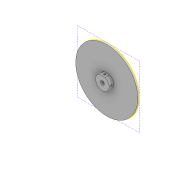
# Autodesk Inventor part: wheel
Saved by Autodesk Inventor 2020 (Build 240168000, 168)
## iProperties
Created: 2021-06-14
Part Number: wheel
Material: Generic
Document SubType Name: Modeling
Designer: Aidan Lee
Density: 1 g/cm^3
Appearance: Default
Author: Aidan Lee
Autodesk Inventor part; units mm, degrees
ref_plane "YZ Plane" through (0, 0, 0) normal (1, 0, 0) x (0, 1, 0)
ref_plane "XZ Plane" through (0, 0, 0) normal (0, 1, 0) x (-1, 0, 0)
ref_plane "XY Plane" through (0, 0, 0) normal (0, 0, 1) x (1, 0, 0)
sketch "Sketch1" plane through (0, 0, 0) normal (0, 0, 1) x (1, 0, 0)
  spline S0 degree 3 poles (-8.9262, 55.5372) (-8.7839, 55.3802) (-8.4991, 55.0662) (-8.0852, 54.5835) (-7.6813, 54.0924) (-7.2889, 53.592) (-6.9084, 53.0826) (-6.5406, 52.5638) (-6.1865, 52.0357) (-5.8469, 51.4981) (-5.5231, 50.9508) (-5.2164, 50.3937) (-4.9286, 49.8267) (-4.6617, 49.2495) (-4.4187, 48.6617) (-4.2033, 48.0633) (-4.0539, 47.5547) (-3.9553, 47.1422) (-3.9241, 46.9325) (-3.9085, 46.8277) knots 0 0 0 0 0.063581 0.127162 0.190743 0.254324 0.317905 0.381486 0.445066 0.508647 0.572227 0.635807 0.699386 0.762964 0.826542 0.890117 0.953687 0.985476 1.017256 1.017256 1.017256 1.017256
  spline S1 degree 3 poles (-3.9085, 46.8277) (-3.8988, 46.6849) (-3.8795, 46.3993) (-3.8286, 45.9728) (-3.7545, 45.5498) (-3.6583, 45.1311) (-3.5319, 44.7205) (-3.3763, 44.3201) (-3.189, 43.9333) (-2.9645, 43.5666) (-2.7433, 43.2845) (-2.5493, 43.0739) (-2.3922, 42.9274) (-2.2262, 42.7911) (-2.0526, 42.6646) (-1.8686, 42.5537) (-1.678, 42.4548) (-1.4812, 42.3683) (-1.2769, 42.302) (-1.0697, 42.2449) (-0.8577, 42.21) (-0.6441, 42.187) (-0.3577, 42.1846) (0, 42.1894) (0.3577, 42.1846) (0.6441, 42.187) (0.8577, 42.21) (1.0697, 42.2449) (1.2769, 42.302) (1.4812, 42.3683) (1.678, 42.4548) (1.8686, 42.5537) (2.0526, 42.6646) (2.2262, 42.7911) (2.3922, 42.9274) (2.5493, 43.0739) (2.7433, 43.2845) (2.9645, 43.5666) (3.189, 43.9333) (3.3763, 44.3201) (3.5319, 44.7205) (3.6583, 45.1311) (3.7545, 45.5498) (3.8286, 45.9728) (3.8795, 46.3993) (3.8988, 46.6849) (3.9085, 46.8277) knots 0 0 0 0 0.04293 0.085861 0.12879 0.17172 0.214646 0.257562 0.300476 0.343394 0.386302 0.407769 0.429238 0.450698 0.472163 0.49363 0.515088 0.536554 0.558017 0.579478 0.600945 0.622403 0.64387 0.686802 0.729734 0.751201 0.772659 0.794126 0.815587 0.83705 0.858516 0.879974 0.901441 0.922906 0.944366 0.965835 0.987302 1.03021 1.073128 1.116042 1.158958 1.201884 1.244814 1.287743 1.330674 1.373604 1.373604 1.373604 1.373604
  spline S2 degree 3 poles (3.9085, 46.8277) (3.9241, 46.9325) (3.9553, 47.1422) (4.0539, 47.5547) (4.2033, 48.0633) (4.4187, 48.6617) (4.6617, 49.2495) (4.9286, 49.8267) (5.2164, 50.3937) (5.5231, 50.9508) (5.8469, 51.4981) (6.1865, 52.0357) (6.5406, 52.5638) (6.9084, 53.0826) (7.2889, 53.592) (7.6813, 54.0924) (8.0852, 54.5835) (8.4991, 55.0662) (8.7839, 55.3802) (8.9262, 55.5372) knots 0 0 0 0 0.03178 0.063568 0.127139 0.190714 0.254291 0.31787 0.381449 0.445029 0.508609 0.572189 0.63577 0.699351 0.762932 0.826513 0.890094 0.953675 1.017256 1.017256 1.017256 1.017256
  circle A0 centre (0, 0) radius 42.1875 construction
  circle A1 centre (0, 0) radius 46.9846 construction
  circle A2 centre (0, 0) radius 50 construction
  circle A3 centre (0, 0) radius 56.25
  point P0 (-8.5013, 55.0643)
  point P1 (-8.0869, 54.5821)
  point P2 (-7.6832, 54.0908)
  point P3 (-7.2909, 53.5905)
  point P4 (-6.9105, 53.081)
  point P5 (-6.5429, 52.5623)
  point P6 (-6.1889, 52.0341)
  point P7 (-5.8496, 51.4965)
  point P8 (-5.526, 50.9492)
  point P9 (-5.2196, 50.3921)
  point P10 (-4.9321, 49.825)
  point P11 (-4.6657, 49.2477)
  point P12 (-4.4233, 48.6599)
  point P13 (-4.2093, 48.0613)
  point P14 (-4.031, 47.4511)
  point P15 (-3.9598, 47.1413)
  point P16 (-3.8758, 46.3996)
  point P17 (-3.8247, 45.9733)
  point P18 (-3.7508, 45.5505)
  point P19 (-3.6533, 45.1324)
  point P20 (-3.527, 44.7221)
  point P21 (-3.371, 44.3223)
  point P22 (-3.1828, 43.9367)
  point P23 (-2.9576, 43.5713)
  point P24 (-2.6935, 43.2332)
  point P25 (-2.5474, 43.0758)
  point P26 (-2.3907, 42.9291)
  point P27 (-2.225, 42.7928)
  point P28 (-2.0509, 42.6672)
  point P29 (-1.8675, 42.5557)
  point P30 (-1.677, 42.4569)
  point P31 (-1.48, 42.3717)
  point P32 (-1.2764, 42.3036)
  point P33 (-1.069, 42.2486)
  point P34 (-0.8574, 42.212)
  point P35 (-0.6439, 42.1905)
  point P36 (-0.4293, 42.1857)
  point P37 (0, 42.1875)
  point P38 (0.4293, 42.1857)
  point P39 (0.6439, 42.1905)
  point P40 (0.8574, 42.212)
  point P41 (1.069, 42.2486)
  point P42 (1.2764, 42.3036)
  point P43 (1.48, 42.3717)
  point P44 (1.677, 42.4569)
  point P45 (1.8675, 42.5557)
  point P46 (2.0509, 42.6672)
  point P47 (2.225, 42.7928)
  point P48 (2.3907, 42.9291)
  point P49 (2.5474, 43.0758)
  point P50 (2.6935, 43.2332)
  point P51 (2.9576, 43.5713)
  point P52 (3.1828, 43.9367)
  point P53 (3.371, 44.3223)
  point P54 (3.527, 44.7221)
  point P55 (3.6533, 45.1324)
  point P56 (3.7508, 45.5505)
  point P57 (3.8247, 45.9733)
  point P58 (3.8758, 46.3996)
  point P59 (3.9598, 47.1413)
  point P60 (4.031, 47.4511)
  point P61 (4.2093, 48.0613)
  point P62 (4.4233, 48.6599)
  point P63 (4.6657, 49.2477)
  point P64 (4.9321, 49.825)
  point P65 (5.2196, 50.3921)
  point P66 (5.526, 50.9492)
  point P67 (5.8496, 51.4965)
  point P68 (6.1889, 52.0341)
  point P69 (6.5429, 52.5623)
  point P70 (6.9105, 53.081)
  point P71 (7.2909, 53.5905)
  point P72 (7.6832, 54.0908)
  point P73 (8.0869, 54.5821)
  point P74 (8.5013, 55.0643)
  constraints: 4 centre point, 2 point on circle, 165 other
extrude "Extrusion1" add sketch "Sketch1" against normal blind 16
extrude "Extrusion2" cut sketch "Sketch1" against normal through all contours A3 S2 S1 S0 picked at (0.9155, 51.5438)
pattern_circular "Circular Pattern1" count 16 over 360 about axis through (0, 0, 0) along (0, 0, -1) of "Extrusion2"
sketch "Measuring" plane through (0, 0, -16) normal (0, 0, -1) x (-1, 0, 0)
  circle A0 centre (0, 0) radius 56.25 projected
  circle A1 centre (0, 0) radius 50
  circle A2 centre (73.063, 68.2774) radius 50 construction
  line L0 (27.9744, 52.4494) -> (54.2214, 24.3627) construction
  line L1 (41.0979, 38.406) -> (73.063, 68.2774) construction
  dimension "d37" = 100
  dimension "d45" = 6.25
  dimension "d46" = 100
  dimension "d47" = 43.75
  constraints: 4 end point, 2 centre point, 1 coincident, 1 equal radius, 1 midpoint, 1 perpendicular, 3 other
  measures "d37" diameter of A1
  measures "d46" diameter of A2
  measures "d47" distance from line of L1.end L0
sketch "Sketch11" plane through (0, 0, 0) normal (1, 0, 0) x (0, 1, 0)
  line L0 (13.8864, 0) -> (-13.8864, 0) construction
  line L1 (-13.8864, 0) -> (-13.8864, -7) construction
  line L2 (-13.8864, -7) -> (13.8864, -7) construction
  line L3 (13.8864, -7) -> (13.8864, 0) construction
  circle A0 centre (0, -3.5) radius 1.5 construction
  line L4 (-1.3941, -2) -> (1.3941, -2) construction
  line L5 (-3.9085, -16) -> (3.9085, -16) construction
  line L6 (-67.1444, 3.8787) -> (73.9482, 3.8787)
  line L7 (73.9482, 3.8787) -> (73.9482, -7)
  line L8 (73.9482, -7) -> (-67.1444, -7)
  line L9 (-67.1444, -7) -> (-67.1444, 3.8787)
  point P0 (0, 0)
  point P1 (0, 0)
  point P2 (-13.8864, -3.5)
  point P3 (0, -2)
  dimension "d48" = 3
  dimension "d49" = 2
  dimension "d50" = 9
  dimension "d58" = 7
  constraints: 18 end point, 4 parallel, 3 horizontal, 3 midpoint, 3 vertical alignment, 2 coincident, 2 perpendicular, 1 collinear, 1 horizontal alignment, 2 other
  measures "d49" distance between parallel lines of L0 L4
  measures "d50" distance between parallel lines of L5 L2
  measures "d58" distance of L2.end L0.start
extrude "Thinner" cut sketch "Sketch11" against normal through all both and the other way through all
sketch "Sketch12" plane through (-16.8651, 41.399, -7) normal (0, 0, 1) x (0.9476, 0.3195, 0)
  circle A0 centre (2.7546, -44.6175) radius 3
  dimension "d54" = 6
  constraints: 1 centre point, 1 coincident
  measures "d54" diameter of A0
extrude "Hole" cut sketch "Sketch12" against normal blind 20
sketch "Sketch13" plane through (-16.8651, 41.399, -7) normal (0, 0, 1) x (0.9476, 0.3195, 0)
  circle A0 centre (2.7546, -44.6175) radius 11
  circle A1 centre (2.7546, -44.6175) radius 3 projected
  dimension "d57" = 8
  constraints: 1 centre point, 1 coincident
  measures "d57" radial gap between concentric circles of A0 A1
extrude "Coupler" add sketch "Sketch13" along normal blind 7
sketch "Sketch14" plane through (-16.8651, 41.399, -7) normal (0, 0, 1) x (0.9476, 0.3195, 0)
  circle A0 centre (11.251, -19.4175) radius 9
  line L0 (16.2331, -4.641) -> (2.7546, -44.6175) construction
  circle A1 centre (2.7546, -44.6175) radius 11 construction
  circle A2 centre (2.7546, -44.6175) radius 11 construction
  line L1 (6.269, -34.194) -> (16.2331, -4.641) construction
  circle A3 centre (-14.821, -24.6594) radius 9
  circle A4 centre (-23.3174, -49.8593) radius 9
  circle A5 centre (-5.7418, -69.8174) radius 9
  circle A6 centre (20.3302, -64.5756) radius 9
  circle A7 centre (28.8266, -39.3756) radius 9
  dimension "d61" = 18
  dimension "d64" = 360
  constraints: 6 centre point, 4 end point, 2 point on line, 1 collinear, 1 midpoint, 15 other
  measures "d61" diameter of A0
extrude "Cutouts" cut sketch "Sketch14" against normal through all
sketch "Sketch15" plane through (0, 0, 0) normal (1, 0, 0) x (0, 1, 0)
  circle A0 centre (0, -3.5) radius 1.5
  line L0 (11, 0) -> (-11, 0) projected
  line L1 (0, 0) -> (0, -7) construction
  line L2 (0, -7) -> (0, 0) construction
  line L3 (-11, -7) -> (11, -7) construction
  point P0 (0, 0)
  point P1 (-10.9663, -7)
  dimension "d68" = 3
  constraints: 4 end point, 2 midpoint, 1 centre point, 1 coincident, 1 collinear, 1 horizontal alignment, 1 point on line, 1 vertical, 1 vertical alignment
  measures "d68" diameter of A0
extrude "SetScrewHole1" cut sketch "Sketch15" along normal through all
sketch "Sketch16" plane through (0, 0, 0) normal (0, 1, 0) x (-1, 0, 0)
  circle A0 centre (0, -3.5) radius 1.5
  line L0 (-11, -7) -> (11, -7) projected
  line L1 (0, 0) -> (0, -7) construction
  dimension "d71" = 3
  constraints: 2 end point, 2 midpoint, 1 centre point, 1 coincident, 1 vertical alignment
  measures "d71" diameter of A0
extrude "Extrusion14" cut sketch "Sketch16" along normal through all
thread "Thread3" size "M3x0.5" class "6H" standard "ANSI Metric M Profile" full length
thread "Thread4" size "M3x0.5" class "6H" standard "ANSI Metric M Profile" full length
sketch "Sketch17" plane through (-16.8651, 41.399, -7) normal (0, 0, 1) x (0.9476, 0.3195, 0)
  line L0 (-62.2572, 14.3784) -> (64.742, 14.3784)
  line L1 (64.742, 14.3784) -> (64.742, -104.7192)
  line L2 (64.742, -104.7192) -> (-62.2572, -104.7192)
  line L3 (-62.2572, -104.7192) -> (-62.2572, 14.3784)
  point P0 (2.7546, -44.6175)
  constraints: 8 end point, 2 parallel, 1 horizontal, 1 perpendicular
extrude "Extrusion15" cut sketch "Sketch17" against normal blind 10
sketch "Sketch18" plane through (0, 0, -7) normal (0, 0, -1) x (-1, 0, 0)
  circle A0 centre (0, 0) radius 50
  dimension "d80" = 100
  constraints: 1 centre point, 1 coincident
  measures "d80" diameter of A0
extrude "Extrusion16" add sketch "Sketch18" along normal blind 3
sketch "Sketch19" plane through (0, 0, -10) normal (0, 0, -1) x (-1, 0, 0)
  line L0 (-50, 50) -> (50, 50) construction
  line L1 (50, 50) -> (50, -50) construction
  line L2 (50, -50) -> (-50, -50) construction
  line L3 (-50, -50) -> (-50, 50) construction
  circle A0 centre (0, 0) radius 50 projected
  constraints: 2 tangent, 2 other
sketch "Sketch20" plane through (0, 0, 0) normal (1, 0, 0) x (0, 1, 0)
  line L0 (-50, -7) -> (50, -7) projected
  line L1 (18.4735, 2.9106) -> (10, 2.9106)
  line L2 (10, 2.9106) -> (10, -7)
  line L3 (10, -7) -> (18.4735, -7)
  line L4 (18.4735, -7) -> (18.4735, 2.9106)
  point P0 (0, 0)
  dimension "d124" = 10
  constraints: 8 end point, 2 parallel, 1 horizontal, 1 perpendicular, 1 point on line
  measures "d124" distance from line of point (0, 0) L2
extrude "Extrusion17" cut sketch "Sketch20" along normal through all both and the other way through all
equation "\"Module\" = 6.25"
equation "\"PressureAngle\" = 20deg"
equation "\"UnitProfileClearance\" = 0.25"
equation "\"UnitRoundRadius\" = 0.35"
equation "\"HeadDiameter\" = 112.5"
equation "\"RootDiameter\" = 84.375"
equation "\"BaseDiameter\" = 93.96926"
equation "\"HelixAngle\" = 0"
equation "\"UnitCorrection\" = 0"
equation "\"UnitAddendumModification\" = 0"
equation "\"CircularPitch\" = 19.634954"
equation "\"UnitBacklashShift\" = 0"
equation "\"TotalToolShift\" = 0"
equation "\"IsInternal\" = 0"
body "Solid1"
